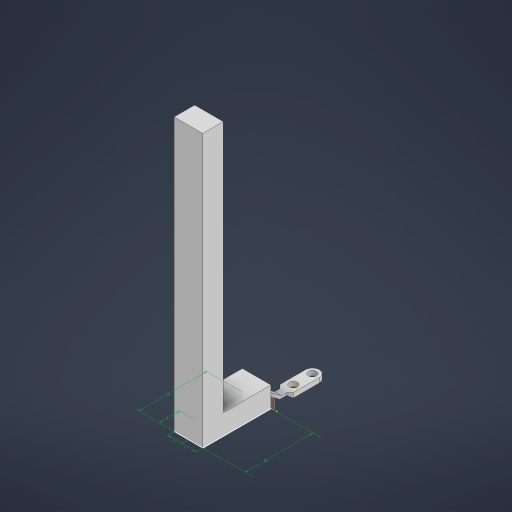
# Autodesk Inventor part: optrode_holder_DG_v2
Saved by Autodesk Inventor 2023 (Build 270158000, 158)
## iProperties
Created: 2022-09-28
Part Number: optrode_holder_DG_v2
Material: Generic
Document SubType Name: Modeling
Designer: c4team_RTX3070
Density: 1 g/cm^3
Appearance: Default
Author: c4team_RTX3070
Autodesk Inventor part; units mm, degrees
ref_plane "YZ Plane" through (0, 0, 0) normal (1, 0, 0) x (0, 1, 0)
ref_plane "XZ Plane" through (0, 0, 0) normal (0, 1, 0) x (-1, 0, 0)
ref_plane "XY Plane" through (0, 0, 0) normal (0, 0, 1) x (1, 0, 0)
sketch "Sketch2" plane through (0, 0, 0) normal (0, 1, 0) x (-1, 0, 0)
  circle A0 centre (1.4547, -3.8269) radius 0.6
  arc A1 (0.4547, -3.8269) -> (2.4547, -3.8269) centre (1.4547, -3.8269) ccw
  circle A2 centre (1.4547, -1.0269) radius 0.6
  line L0 (2.4547, -3.8269) -> (2.4547, -1.0269)
  line L1 (0.4547, -1.0269) -> (0.4547, -3.8269)
  line L2 (2.4547, -1.0269) -> (2.4547, -0.0269)
  line L3 (2.4547, -0.0269) -> (0.4547, -0.0269)
  line L4 (0.4547, -0.0269) -> (0.4547, -1.0269)
  line L5 (2.4547, -0.0269) -> (1.4547, -0.0269)
  line L6 (1.4547, -0.0269) -> (0.9547, -0.0269)
  line L7 (0.9547, -0.0269) -> (0.9547, 0.9731)
  line L8 (1.4547, -0.0269) -> (1.9547, -0.0269)
  line L9 (1.9547, -0.0269) -> (1.9547, 0.9731)
  line L10 (1.9547, 0.9731) -> (0.9547, 0.9731)
  dimension "d37" = 1.2
  dimension "d38" = 2
  dimension "d39" = 1.2
  dimension "d42" = 2.8
  dimension "d43" = 1
  dimension "d47" = 1
  constraints: 22 end point, 4 horizontal, 3 centre point, 3 perpendicular, 2 collinear, 2 point on circle, 1 coincident, 1 tangent, 1 vertical
  measures "d37" diameter of A0
  measures "d38" diameter of A1
  measures "d39" diameter of A2
  measures "d42" distance of A2.centre A0.centre
  measures "d43" distance of L0.end L2.end
  measures "d47" distance of L6.end L7.end
extrude "Extrusion5" add sketch "Sketch2" along normal blind 0.7 contours L1 L4 L3 L2 L0 A1
sketch "Sketch14" plane through (-2.4547, 0, -0.0269) normal (0, 0, 1) x (1, 0, 0)
  line L0 (0, 0.7) -> (2, 0.7) projected
  line L1 (1, 0.7) -> (1.5166, 0.7)
  line L2 (1.5166, 0.7) -> (1.5166, 0.35)
  line L3 (0.5166, 0.35) -> (0.5166, 0.7)
  line L4 (0.5166, 0.7) -> (1.0166, 0.7)
  line L5 (0.5166, 0.35) -> (1.5166, 0.35)
  point P0 (2.4547, 0)
  point P1 (0.5166, 0.525)
  dimension "d84" = 0.35
  constraints: 10 end point, 2 horizontal, 2 midpoint, 1 perpendicular, 1 point on line
  measures "d84" distance of L2.end L1.end
extrude "Extrusion12" add sketch "Sketch14" along normal blind 0.5
loft "Loft1" add section 1 edges at (-0.9381, 0.525, 0.4731) (-1.4381, 0.7, 0.4731) (-1.9381, 0.525, 0.4731) (-1.4381, 0.35, 0.4731) section 2 edges at (-1.9381, 0.525, -0.0269) (-2.1964, 0.7, -0.0269) (-2.4547, 0.35, -0.0269) (-1.4547, 0, -0.0269) (-0.4547, 0.35, -0.0269) (-0.6964, 0.7, -0.0269) (-0.9381, 0.525, -0.0269) (-1.4381, 0.35, -0.0269)
sketch "Sketch15" plane through (-2.4547, 0, 0.4731) normal (0, 0, 1) x (1, 0, 0)
  line L0 (0.5166, 0.7) -> (0.5166, 0.35) projected
  line L1 (0.4, 0.7) -> (1.6, 0.7) projected
  line L2 (0.5166, 0.35) -> (1.5166, 0.35)
  line L3 (1.5166, 0.35) -> (1.5166, 0.7)
  line L4 (1.5166, 0.7) -> (0.5166, 0.7)
  line L5 (0.5166, 0.7) -> (0.5166, 0.35)
  point P0 (2.4547, 0)
  dimension "d92" = 1
  constraints: 8 end point, 2 parallel, 1 horizontal, 1 perpendicular, 1 point on line
  measures "d92" distance of L4.end L3.end
extrude "Extrusion13" add sketch "Sketch15" along normal blind 1
ref_plane "Work Plane3" through (-1.6881, 1.4071, 2.8802) normal (0, 0, 1) x (1, 0, 0)
sketch "Sketch19" plane through (-1.6881, 1.4071, 2.8802) normal (0, 0, 1) x (1, 0, 0)
  line L0 (-0.25, 0) -> (0.75, 0) projected
  line L1 (0.75, 0) -> (-0.2653, 0)
  line L2 (-0.2653, 0) -> (-0.2653, 0.5)
  line L3 (-0.2653, 0.5) -> (0.75, 0.5)
  line L4 (0.75, 0.5) -> (0.75, 0)
  point P0 (1.6881, -1.4071)
  dimension "d102" = 0.5
  constraints: 8 end point, 2 parallel, 1 horizontal, 1 perpendicular
  measures "d102" distance of L1.end L2.end
extrude "Extrusion16" add sketch "Sketch19" along normal blind 0.5
sketch "Sketch20" plane through (-1.6881, 1.4071, 3.3802) normal (0, 0, 1) x (1, 0, 0)
  line L0 (0.75, 0.5) -> (-0.2653, 0.5) projected
  line L1 (-0.2653, 0.5) -> (-0.2653, 0) projected
  line L2 (0.75, 0.5) -> (-0.2653, 0.5)
  line L3 (-0.2653, 0.5) -> (-0.2653, 0)
  line L4 (-0.2653, 0) -> (0.75, 0)
  line L5 (0.75, 0) -> (0.75, 0.5)
  point P0 (1.6881, -1.4071)
  constraints: 8 end point, 2 parallel, 1 horizontal, 1 perpendicular
extrude "Extrusion17" add sketch "Sketch20" along normal blind 1
sketch "Sketch21" plane through (-1.9534, 1.4071, 2.8802) normal (0, -1, 0) x (1, 0, 0)
  line L0 (1.0153, 1.5) -> (0, 1.5) projected
  line L1 (0.5077, 1.5) -> (-1.5923, 1.5)
  line L2 (-1.5923, 1.5) -> (-1.5923, 11.5)
  line L3 (-1.5923, 11.5) -> (0.5077, 11.5)
  line L4 (0.5077, 11.5) -> (0.5077, 1.5)
  line L5 (0.5077, 1.5) -> (2.6077, 1.5)
  line L6 (2.6077, 1.5) -> (2.6077, 11.5)
  line L7 (2.6077, 11.5) -> (0.5077, 11.5)
  line L8 (0.5077, 11.5) -> (0.5077, 1.5)
  line L9 (2.6077, 8.5) -> (-1.5923, 8.5)
  point P0 (1.9534, -2.8802)
  point P1 (1.0153, 1.5)
  point P2 (0.5077, 11.5)
  dimension "d111" = 2.1
  dimension "d112" = 2.1
  dimension "d113" = 10
  dimension "d114" = 10
  dimension "d115" = 3
  constraints: 18 end point, 4 parallel, 3 perpendicular, 2 horizontal, 2 point on line, 1 midpoint
  measures "d111" distance of L6.end L7.end
  measures "d112" distance of L2.end L3.end
  measures "d113" distance of L1.end L2.end
  measures "d114" distance of L5.end L6.end
  measures "d115" distance between parallel lines of L3 L9
extrude "Extrusion18" add sketch "Sketch21" against normal blind 3 contours L0 L4 L9 L6 L5 | L0 L1 L2 L9 L4
extrude "Extrusion19" add sketch "Sketch21" against normal blind 40 contours L9 L2 L3 L4 | L4 L7 L6 L9
sketch "Sketch23" plane through (-1.6881, 1.4071, 2.8802) normal (0, 0, 1) x (1, 0, 0)
  point P0 (1.6881, -1.4071)
sketch "Sketch24" plane through (-1.6881, 1.4071, 2.8802) normal (0, 0, 1) x (1, 0, 0)
  point P0 (1.6881, -1.4071)
sketch "Sketch25" plane through (-0.9381, 0.35, 0.4731) normal (1, 0, 0) x (0, 0, -1)
  point P0 (0.4731, -0.35)
draft "FaceDraft6" angle -30 pull direction (0, -1, 0) faces at (-1.2714, 0.4667, 1.4731) fixed edges at (-1.4381, 0.35, 1.4731)
loft "Loft4" add section 1 edges at (-1.4457, 1.9071, 2.8802) (-0.9381, 1.6571, 2.8802) (-1.4457, 1.4071, 2.8802) (-1.9534, 1.6571, 2.8802) section 2 edges at (-0.9381, 0.525, 1.3721) (-1.4381, 0.7, 1.2711) (-1.9381, 0.525, 1.3721) (-1.4381, 0.35, 1.4731)
body "Solid2"
